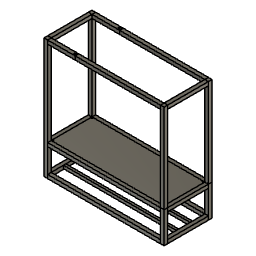
KUKA bur første utkast forbedret v6 (Autodesk Fusion 360 design; units mm, degrees)
Autodesk Fusion 360 part; units mm, degrees
note: some values were not read from the file. Set by a fixed rule: which sketch regions a step uses.
sketch "Hovedtegning" plane through (0, 0, 0) normal (0, 0, 1) x (1, 0, 0)
  line L0 (1000, 400) -> (-1000, 400)
  line L1 (-1000, 400) -> (-1000, -400)
  line L2 (-1000, -400) -> (1000, -400)
  line L3 (1000, -400) -> (1000, 400)
  line L4 (1000, 400) -> (-1000, -400) construction
  line L5 (-1000, 400) -> (1000, -400) construction
  line L6 (940, -340) -> (-940, -340)
  line L7 (-940, -340) -> (-940, 340)
  line L8 (-940, 340) -> (940, 340)
  line L9 (940, 340) -> (940, -340)
  line L10 (940, -340) -> (-940, 340) construction
  line L11 (-940, -340) -> (940, 340) construction
  line L12 (-1000, -400) -> (-940, -400)
  line L13 (-940, -400) -> (-940, -340)
  line L14 (-940, -340) -> (-1000, -340)
  line L15 (-1000, -340) -> (-1000, -400)
  line L16 (-1000, 400) -> (-940, 400)
  line L17 (-940, 400) -> (-940, 340)
  line L18 (-940, 340) -> (-1000, 340)
  line L19 (-1000, 340) -> (-1000, 400)
  line L20 (940, 340) -> (1000, 340)
  line L21 (1000, 340) -> (1000, 400)
  line L22 (1000, 400) -> (940, 400)
  line L23 (940, 400) -> (940, 340)
  line L24 (940, -340) -> (1000, -340)
  line L25 (1000, -340) -> (1000, -400)
  line L26 (1000, -400) -> (940, -400)
  line L27 (940, -400) -> (940, -340)
  dimension "d4" = 2000
  dimension "d5" = 800
  dimension "d6" = 680
  dimension "d7" = 1880
  constraint perpendicular L0 L1
  constraint parallel L0 L2
  constraint parallel L1 L3
  constraint horizontal L0
  constraint coincident L4 origin
  constraint coincident L5 origin
  constraint perpendicular L6 L7
  constraint parallel L6 L8
  constraint parallel L7 L9
  constraint horizontal L6
  constraint coincident L10 origin
  constraint coincident L11 origin
  constraint horizontal L12
  constraint vertical L13
  constraint horizontal L14
  constraint vertical L15
  constraint horizontal L16
  constraint vertical L17
  constraint horizontal L18
  constraint vertical L19
  constraint horizontal L20
  constraint vertical L21
  constraint horizontal L22
  constraint vertical L23
  constraint horizontal L24
  constraint vertical L25
  constraint horizontal L26
  constraint vertical L27
  measures "d4" distance of L1.end L2.end
  measures "d5" distance of L0.end L1.end
  measures "d6" distance of L6.end L7.end
  measures "d7" distance of L7.end L8.end
extrude "Extrude1" add sketch "Hovedtegning" along normal blind 2000 contours L1 L2 L12 L13 L14 L15 makes body 1
extrude "Extrude2" add sketch "Hovedtegning" along normal blind 2000 separate body contours L0 L1 L16 L17 L18 L19 makes body 2
extrude "Extrude3" add sketch "Hovedtegning" along normal blind 520 separate body contours L0 L3 L20 L21 L22 L23 | L2 L3 L24 L25 L26 L27 makes body 3 at (960, 340, 173.3333) makes body 4 at (960, -400, 173.3333)
extrude "Extrude4" add sketch "Hovedtegning" along normal blind 60 separate body contours L1 L7 L14 L18 makes body 5
extrude "Extrude5" add sketch "Hovedtegning" along normal blind 60 separate body contours L2 L6 L13 L27 makes body 6
extrude "Extrude6" add sketch "Hovedtegning" along normal blind 60 separate body contours L0 L8 L17 L23 makes body 7
extrude "Extrude7" add sketch "Hovedtegning" along normal blind 60 separate body contours L3 L9 L20 L24 makes body 8
ref_plane "WorkPlane1" through (0, 0, 460) normal (0, 0, 1) x (1, 0, 0)
sketch "Plate utvendig" plane through (0, 0, 460) normal (0, 0, 1) x (1, 0, 0)
  line L0 (-1000, 400) -> (1000, 400)
  line L1 (1000, 400) -> (1000, -400)
  line L2 (1000, -400) -> (-1000, -400)
  line L3 (-1000, -400) -> (-1000, 400)
  line L4 (-1000, 400) -> (1000, -400) construction
  line L5 (1000, 400) -> (-1000, -400) construction
  dimension "d24" = 2000
  dimension "d25" = 800
  constraint perpendicular L0 L1
  constraint parallel L0 L2
  constraint parallel L1 L3
  constraint horizontal L0
  constraint coincident L4 origin
  constraint coincident L5 origin
  measures "d24" distance of L1.end L2.end
  measures "d25" distance of L0.end L1.end
sketch "Plate innvendig" plane through (0, 0, 460) normal (0, 0, 1) x (1, 0, 0)
  line L0 (940, 340) -> (-940, 340)
  line L1 (-940, 340) -> (-940, -340)
  line L2 (-940, -340) -> (940, -340)
  line L3 (940, -340) -> (940, 340)
  line L4 (940, 340) -> (-940, -340) construction
  line L5 (-940, 340) -> (940, -340) construction
  dimension "d27" = 1880
  dimension "d28" = 680
  constraint perpendicular L0 L1
  constraint parallel L0 L2
  constraint parallel L1 L3
  constraint horizontal L0
  constraint coincident L4 origin
  constraint coincident L5 origin
  measures "d27" distance of L1.end L2.end
  measures "d28" distance of L0.end L1.end
sketch "Sketch4" plane through (0, 0, 460) normal (0, 0, 1) x (1, 0, 0)
  line L0 (-1000, -400) -> (-940, -400)
  line L1 (-940, -400) -> (-940, -340)
  line L2 (-940, -340) -> (-1000, -340)
  line L3 (-1000, -340) -> (-1000, -400)
  line L4 (1000, -400) -> (940, -400)
  line L5 (940, -400) -> (940, -340)
  line L6 (940, -340) -> (1000, -340)
  line L7 (1000, -340) -> (1000, -400)
  line L8 (1000, 400) -> (940, 400)
  line L9 (940, 400) -> (940, 340)
  line L10 (940, 340) -> (1000, 340)
  line L11 (1000, 340) -> (1000, 400)
  line L12 (-1000, 400) -> (-940, 400)
  line L13 (-940, 400) -> (-940, 340)
  line L14 (-940, 340) -> (-1000, 340)
  line L15 (-1000, 340) -> (-1000, 400)
  dimension "d29" = 60
  dimension "d30" = 60
  constraint horizontal L0
  constraint vertical L1
  constraint horizontal L2
  constraint vertical L3
  constraint horizontal L4
  constraint vertical L5
  constraint horizontal L6
  constraint vertical L7
  constraint horizontal L8
  constraint vertical L9
  constraint horizontal L10
  constraint vertical L11
  constraint horizontal L12
  constraint vertical L13
  constraint horizontal L14
  constraint vertical L15
  measures "d29" distance of L4.start L4.end
  measures "d30" distance of L4.start L6.end
sketch "Plate kanter" plane through (0, 0, 460) normal (0, 0, 1) x (1, 0, 0)
  line L0 (-1000, 340) -> (-940, 340)
  line L1 (-940, 340) -> (-940, -340)
  line L2 (-940, -340) -> (-1000, -340)
  line L3 (-1000, -340) -> (-1000, 340)
  line L4 (-940, -340) -> (940, -340)
  line L5 (940, -340) -> (940, -400)
  line L6 (940, -400) -> (-940, -400)
  line L7 (-940, -400) -> (-940, -340)
  line L8 (1000, -340) -> (940, -340)
  line L9 (940, -340) -> (940, 340)
  line L10 (940, 340) -> (1000, 340)
  line L11 (1000, 340) -> (1000, -340)
  line L12 (940, 400) -> (-940, 400)
  line L13 (-940, 400) -> (-940, 340)
  line L14 (-940, 340) -> (940, 340)
  line L15 (940, 340) -> (940, 400)
  constraint horizontal L0
  constraint vertical L1
  constraint horizontal L2
  constraint vertical L3
  constraint horizontal L4
  constraint vertical L5
  constraint horizontal L6
  constraint vertical L7
  constraint horizontal L8
  constraint vertical L9
  constraint horizontal L10
  constraint vertical L11
  constraint horizontal L12
  constraint vertical L13
  constraint horizontal L14
  constraint vertical L15
extrude "Extrude8" add sketch "Plate kanter" along normal blind 60 separate body contours L0 L1 L2 L3 | L12 L13 L14 L15 | L4 L5 L6 L7 | L8 L9 L10 L11 makes body 9 at (940, -113.3333, 480)
ref_plane "WorkPlane2" through (0, 0, 1940) normal (0, 0, 1) x (1, 0, 0)
sketch "Kontrollboks profiler" plane through (-940, 0, 0) normal (1, 0, 0) x (0, 1, 0)
  line L0 (-340, 0) -> (340, 0)
  line L1 (340, 0) -> (340, 60)
  line L2 (-340, 60) -> (-340, 0)
  line L3 (-95, 10) -> (-135, 10)
  line L4 (-135, 10) -> (-135, 60)
  line L5 (-135, 60) -> (-95, 60)
  line L6 (-95, 60) -> (-95, 10)
  line L7 (-95, 10) -> (-135, 60) construction
  line L8 (-135, 10) -> (-95, 60) construction
  line L9 (135, 10) -> (95, 10)
  line L10 (95, 10) -> (95, 60)
  line L11 (95, 60) -> (135, 60)
  line L12 (135, 60) -> (135, 10)
  line L13 (135, 10) -> (95, 60) construction
  line L14 (95, 10) -> (135, 60) construction
  point P0 (-115, 35)
  point P1 (115, 35)
  constraint perpendicular L3 L4
  constraint parallel L3 L5
  constraint parallel L4 L6
  constraint horizontal L3
  constraint coincident L7 P0
  constraint coincident L8 P0
  constraint perpendicular L9 L10
  constraint parallel L9 L11
  constraint parallel L10 L12
  constraint horizontal L9
  constraint coincident L13 P1
  constraint coincident L14 P1
extrude "Extrude10" add sketch "Kontrollboks profiler" along normal blind 1880 separate body contours L9 L10 L11 L12 makes body 10
extrude "Extrude9" add sketch "Kontrollboks profiler" along normal blind 1880 separate body contours L3 L4 L5 L6 makes body 11
sketch "Lengde topp profiler" plane through (-940, 0, 0) normal (1, 0, 0) x (0, 1, 0)
  line L0 (-400, 0) -> (-340, 0)
  line L1 (-340, 2000) -> (-400, 2000)
  line L2 (-400, 2000) -> (-340, 2000)
  line L3 (-340, 2000) -> (-340, 1940)
  line L4 (-340, 1940) -> (-400, 1940)
  line L5 (-400, 1940) -> (-400, 2000)
  line L6 (340, 2000) -> (400, 2000)
  line L7 (400, 2000) -> (400, 1940)
  line L8 (400, 1940) -> (340, 1940)
  line L9 (340, 1940) -> (340, 2000)
  constraint horizontal L2
  constraint vertical L3
  constraint horizontal L4
  constraint vertical L5
  constraint coincident L1.end L2.start
  constraint horizontal L6
  constraint vertical L7
  constraint horizontal L8
  constraint vertical L9
sketch "Bredde topp profiler" plane through (0, 340, 0) normal (0, -1, 0) x (1, 0, 0)
  line L0 (-1000, 0) -> (-940, 0)
  line L1 (-940, 2000) -> (-1000, 2000)
  line L2 (-1000, 2000) -> (-940, 2000)
  line L3 (-940, 2000) -> (-940, 1940)
  line L4 (-940, 1940) -> (-1000, 1940)
  line L5 (-1000, 1940) -> (-1000, 2000)
  line L6 (940, 2000) -> (1000, 2000)
  line L7 (1000, 2000) -> (1000, 1940)
  line L8 (1000, 1940) -> (940, 1940)
  line L9 (940, 1940) -> (940, 2000)
  constraint horizontal L2
  constraint vertical L3
  constraint horizontal L4
  constraint vertical L5
  constraint coincident L1.end L2.start
  constraint horizontal L6
  constraint vertical L7
  constraint horizontal L8
  constraint vertical L9
extrude "Extrude11" add sketch "Bredde topp profiler" along normal blind 680 separate body contours L1 L2 L3 L4 L5 makes body 12
extrude "Extrude12" add sketch "Bredde topp profiler" along normal blind 680 separate body contours L6 L7 L8 L9 makes body 13
extrude "Extrude13" add sketch "Lengde topp profiler" along normal blind 460 separate body contours L1 L2 L3 L4 L5 makes body 14
extrude "Extrude14" add sketch "Lengde topp profiler" along normal blind 460 separate body contours L6 L7 L8 L9 makes body 15
sketch "Plate kanter (1)" plane through (0, 0, 460) normal (0, 0, 1) x (1, 0, 0)
  line L0 (940, -340) -> (1000, -340)
  line L1 (1000, -340) -> (1000, -400)
  line L2 (1000, -400) -> (940, -400)
  line L3 (940, -400) -> (940, -340)
  line L4 (940, 400) -> (1000, 400)
  line L5 (1000, 400) -> (1000, 340)
  line L6 (1000, 340) -> (940, 340)
  line L7 (940, 340) -> (940, 400)
  line L8 (-940, 400) -> (-1000, 400)
  line L9 (-1000, 400) -> (-1000, 340)
  line L10 (-1000, 340) -> (-940, 340)
  line L11 (-940, 340) -> (-940, 400)
  line L12 (-940, -340) -> (-1000, -340)
  line L13 (-1000, -340) -> (-1000, -400)
  line L14 (-1000, -400) -> (-940, -400)
  line L15 (-940, -400) -> (-940, -340)
  constraint horizontal L0
  constraint vertical L1
  constraint horizontal L2
  constraint vertical L3
  constraint horizontal L4
  constraint vertical L5
  constraint horizontal L6
  constraint vertical L7
  constraint horizontal L8
  constraint vertical L9
  constraint horizontal L10
  constraint vertical L11
  constraint horizontal L12
  constraint vertical L13
  constraint horizontal L14
  constraint vertical L15
ref_plane "WorkPlane3" through (0, 0, 520) normal (0, 0, 1) x (1, 0, 0)
sketch "Sketch12" plane through (0, 0, 520) normal (0, 0, 1) x (1, 0, 0)
  line L0 (940, 340) -> (-940, 340)
  line L1 (-940, 340) -> (-940, -340)
  line L2 (-940, -340) -> (940, -340)
  line L3 (940, -340) -> (940, 340)
  constraint horizontal L0
  constraint vertical L1
  constraint horizontal L2
  constraint vertical L3
extrude "Extrude15" add sketch "Sketch12" against normal blind 20 separate body makes body 16
sketch "Sketch13" plane through (0, 0, 520) normal (0, 0, 1) x (-1, 0, 0)
  line L0 (-940, 340) -> (-940, -340)
  line L1 (-940, -340) -> (940, -340)
  line L2 (940, -340) -> (940, 340)
  line L3 (940, 340) -> (-940, 340)
sketch "Sketch15" plane through (0, 0, 520) normal (0, 0, 1) x (-1, 0, 0)
  circle A0 centre (940, -340) radius 30
  circle A1 centre (-940, -340) radius 30
  circle A2 centre (-940, 340) radius 30
  circle A3 centre (940, 340) radius 30
  dimension "d55" = 60
  dimension "d56" = 60
  dimension "d57" = 60
  dimension "d58" = 60
  measures "d55" diameter of A0
  measures "d56" diameter of A1
  measures "d57" diameter of A2
  measures "d58" diameter of A3
extrude "Extrude16" cut sketch "Sketch15" against normal blind 100 bodies 16
sketch "Sketch25" plane through (940, 0, 0) normal (-1, 0, 0) x (0, -1, 0)
  line L0 (-400, 0) -> (-340, 0)
  line L1 (-340, 0) -> (-340, 520)
  line L2 (-340, 520) -> (-400, 520)
  line L3 (-400, 520) -> (-400, 0)
  line L4 (-400, 520) -> (-340, 520)
  line L5 (-340, 520) -> (-340, 460)
  line L6 (-340, 460) -> (-400, 460)
  line L7 (-400, 460) -> (-400, 520)
  line L8 (340, 2000) -> (400, 2000)
  line L9 (400, 2000) -> (400, 1940)
  line L10 (400, 1940) -> (340, 1940)
  line L11 (340, 1940) -> (340, 2000)
  constraint horizontal L4
  constraint vertical L5
  constraint horizontal L6
  constraint vertical L7
  constraint coincident L1 L5.end
  constraint coincident L2.end L3.start
  constraint horizontal L8
  constraint vertical L9
  constraint horizontal L10
  constraint vertical L11
extrude "Extrude18" add sketch "Sketch25" along normal blind 1420 separate body contours L8 L9 L10 L11 makes body 17
sketch "Sketch26" plane through (-480, 0, 0) normal (1, 0, 0) x (0, 1, 0)
  line L0 (340, 1940) -> (400, 1940)
  line L1 (400, 1940) -> (400, 2000)
  line L2 (400, 2000) -> (340, 2000)
  line L3 (340, 2000) -> (340, 1940)
  line L4 (340, 2000) -> (400, 2000)
  line L5 (400, 2000) -> (400, 1940)
  line L6 (400, 1940) -> (340, 1940)
  line L7 (340, 1940) -> (340, 2000)
  constraint horizontal L4
  constraint vertical L5
  constraint horizontal L6
  constraint vertical L7
  constraint coincident L0.end L1.start
  constraint coincident L2.end L3.start
extrude "Extrude19" add sketch "Sketch26" along normal blind 1420 separate body makes body 18
sketch "Hengsel profil" plane through (0, 0, 520) normal (0, 0, 1) x (-1, 0, 0)
  line L0 (-940, 400) -> (-1000, 400)
  line L1 (-1000, 400) -> (-1000, 340)
  line L2 (-1000, 340) -> (-940, 340)
  line L3 (-940, 340) -> (-940, 400)
  line L4 (-940, 340) -> (-1000, 340)
  line L5 (-1000, 340) -> (-1000, 400)
  line L6 (-1000, 400) -> (-940, 400)
  line L7 (-940, 400) -> (-940, 340)
  line L8 (-940, -400) -> (-1000, -400)
  line L9 (-1000, -400) -> (-1000, -340)
  line L10 (-1000, -340) -> (-940, -340)
  line L11 (-940, -340) -> (-940, -400)
  constraint horizontal L4
  constraint vertical L5
  constraint horizontal L6
  constraint vertical L7
  constraint coincident L0.end L1.start
  constraint coincident L2.end L3.start
  constraint horizontal L8
  constraint vertical L9
  constraint horizontal L10
  constraint vertical L11
extrude "Extrude20" add sketch "Hengsel profil" along normal blind 1480 separate body contours L0 L1 L2 L3 L4 L5 L6 L7 makes body 19
extrude "Extrude21" add 1 faces at (980, 360, 520) along direction (0, 0, 1) blind 1480 separate body on bodies 3 makes body 20
sketch "Sketch28" plane through (0, 0, 2000) normal (0, 0, 1) x (-1, 0, 0)
  line L0 (-940, 400) -> (-940, 340)
  line L1 (-940, 340) -> (480, 340)
  line L2 (480, 340) -> (480, 400)
  line L3 (480, 400) -> (-940, 400)
  line L4 (435, 385) -> (525, 385)
  line L5 (525, 385) -> (525, 355)
  line L6 (525, 355) -> (435, 355)
  line L7 (435, 355) -> (435, 385)
  line L8 (435, 385) -> (525, 355) construction
  line L9 (525, 385) -> (435, 355) construction
  point P0 (480, 370)
  dimension "d75" = 90
  dimension "d76" = 30
  constraint perpendicular L4 L5
  constraint parallel L4 L6
  constraint parallel L5 L7
  constraint horizontal L4
  constraint coincident L8 P0
  constraint coincident L9 P0
  constraint midpoint L2 P0
  measures "d75" distance of L5.end L6.end
  measures "d76" distance of L4.end L5.end
extrude "Extrude22" cut sketch "Sketch28" against normal blind 30 contours L2 L4 L5 L6 bodies 14
sketch "Sketch29" plane through (0, 0, 1970) normal (0, 0, 1) x (-1, 0, 0)
  line L0 (525, 355) -> (525, 385)
  line L1 (525, 385) -> (480, 385)
  line L2 (480, 385) -> (480, 355)
  line L3 (480, 355) -> (525, 355)
  line L4 (502.5, 355) -> (480, 355)
  line L5 (480, 355) -> (480, 385)
  line L6 (480, 385) -> (502.5, 385)
  line L7 (502.5, 385) -> (502.5, 355)
  constraint horizontal L4
  constraint vertical L5
  constraint horizontal L6
  constraint vertical L7
  constraint coincident L1.end L2.start
  constraint midpoint L3 L4.start
extrude "Extrude23" add sketch "Sketch29" along normal blind 15 contours L1 L2 L3 L4 L5 L6 L7 bodies 14
move_face "MoveFace1" to x (0.906308, 0, 0.422618) y (0, 1, 0) z (-0.422618, 0, 0.906308) at (792.9881, 0, 393.062) 1 faces at (-487.5, -365, 1985) on bodies 14
sketch "Sketch30" plane through (0, 0, 2000) normal (0, 0, 1) x (-1, 0, 0)
  line L0 (480, -400) -> (480, -340)
  line L1 (480, -340) -> (-940, -340)
  line L2 (-940, -340) -> (-940, -400)
  line L3 (-940, -400) -> (480, -400)
  line L4 (435, -355) -> (525, -355)
  line L5 (525, -355) -> (525, -385)
  line L6 (525, -385) -> (435, -385)
  line L7 (435, -385) -> (435, -355)
  line L8 (435, -355) -> (525, -385) construction
  line L9 (525, -355) -> (435, -385) construction
  line L10 (480, -385) -> (502.5, -385)
  line L11 (502.5, -355) -> (480, -355)
  line L12 (480, -355) -> (480, -385)
  point P0 (480, -370)
  dimension "d82" = 30
  dimension "d83" = 90
  dimension "d84" = 22.5
  constraint perpendicular L4 L5
  constraint parallel L4 L6
  constraint parallel L5 L7
  constraint horizontal L4
  constraint coincident L8 P0
  constraint coincident L9 P0
  constraint midpoint L0 P0
  constraint horizontal L10
  constraint horizontal L11
  constraint vertical L12
  constraint midpoint L6 L10.start
  measures "d82" distance of L4.end L5.end
  measures "d83" distance of L5.end L6.end
  measures "d84" distance of L10.start L10.end
extrude "Extrude25" cut sketch "Sketch30" against normal blind 30 contours L0 L4 L5 L6 L10 L11 L12 bodies 15
sketch "Sketch31" plane through (0, 0, 1970) normal (0, 0, 1) x (-1, 0, 0)
  line L0 (525, -355) -> (480, -355)
  line L1 (480, -355) -> (480, -385)
  line L2 (480, -385) -> (525, -385)
  line L3 (525, -385) -> (525, -355)
  line L4 (480, -385) -> (502.5, -385)
  line L5 (502.5, -385) -> (502.5, -355)
  line L6 (502.5, -355) -> (480, -355)
  line L7 (480, -355) -> (480, -385)
  constraint horizontal L4
  constraint vertical L5
  constraint horizontal L6
  constraint vertical L7
  constraint midpoint L0 L5.end
  constraint coincident L1.end L2.start
extrude "Extrude26" add sketch "Sketch31" along normal blind 15 contours L0 L1 L2 L4 L5 L6 L7 bodies 15
move_face "MoveFace2" to x (0.866025, 0, 0.5) y (0, 1, 0) z (-0.5, 0, 0.866025) at (926.685, 0, 511.5646) 1 faces at (-487.5, 365, 1985) on bodies 15
equation "Lengde = 2000 mm"
equation "Bredde = 800 mm"
equation "Høyde = 2000 mm"
equation "d4 = Lengde"
equation "d5 = Bredde"
equation "d6 = Bredde - 120 mm"
equation "d7 = Lengde - 120 mm"
equation "d8 = Høyde"
equation "d10 = Høyde"
equation "Profil = 60 mm"
equation "d15 = Profil"
equation "d17 = Profil"
equation "d19 = Profil"
equation "d21 = Profil"
equation "d24 = Lengde"
equation "d25 = Bredde"
equation "PlateTykkelse = 200 mm"
equation "d27 = Lengde - 120 mm"
equation "d28 = Bredde - 120 mm"
equation "d31 = Profil"
equation "d33 = Høyde - 60 mm"
equation "d40 = Bredde - 120 mm"
equation "d42 = Bredde - 120 mm"
equation "d71 = Høyde - 520 mm"
equation "d73 = Høyde - 520 mm"
named bodies: "Venstre fot1", "Venstre fot2", "Høyre fot2", "Høyre fot1", "Høyre bunn", "Bak bunn", "Foran bunn", "Venstre bunn", "Plate kanter", "Foran kontrollboksprofil", "Bak kontrollboksprofil", "Venstre øvreprofil", "Høyre øvreprofil", "Foran venstre øvreprofil", "Bak venstre øvreprofil", "Plate", "Foran høyre øvreprofil", "Bak høyre øvreprofil", "Foran hengselprofil", "Bak hengselprofil"
